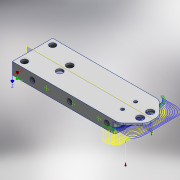
# Autodesk Inventor part: c-head-flange
Saved by Autodesk Inventor 2016 (Build 200138000, 138)
## iProperties
Created: 2015-05-12
Part Number: c-head-flange
Material: Aluminum 6061
Document SubType Name: Modeling
Designer: as
Mass: 10.115 g
Surface Area: 39.4991 cm^2
Volume: 3.74628 cm^3
Density: 2.7 g/cm^3
Appearance: Aluminum - Flat
Author: as
Autodesk Inventor part; units mm, degrees
ref_plane "YZ Plane" through (0, 0, 0) normal (1, 0, 0) x (0, 1, 0)
ref_plane "XZ Plane" through (0, 0, 0) normal (0, 1, 0) x (-1, 0, 0)
ref_plane "XY Plane" through (0, 0, 0) normal (0, 0, 1) x (1, 0, 0)
sketch "Sketch1" plane through (0, 0, 0) normal (0, 0, 1) x (1, 0, 0)
  line L0 (-6, -20) -> (60, -20)
  line L1 (60, -20) -> (60, 0)
  line L2 (60, 0) -> (-6, 0)
  line L3 (-6, 0) -> (-6, -20)
  point P0 (0, 0)
  dimension "d2" = 20
  dimension "d3" = 66
  dimension "d8" = 60
  dimension "d9" = 0
  constraints: 8 end point, 2 parallel, 1 horizontal, 1 perpendicular
  measures "d2" distance of L0.end L1.end
  measures "d3" distance of L1.end L2.end
  measures "d8" distance from line of point (0, 0) L1
  measures "d9" distance from line of point (0, 0) L2
extrude "Extrusion1" add sketch "Sketch1" along normal blind 6
sketch "Sketch5" plane through (0, 0, 6) normal (0, 0, 1) x (1, 0, 0)
  line L0 (-6, 0) -> (-6, -20) projected
  point P0 (0, 0)
  point P1 (-3, -3)
  point P2 (-3, -17)
  dimension "d48" = 3
  dimension "d50" = 17
  dimension "d51" = 3
  dimension "d53" = 3
  measures "d48" horizontal distance of L0.start point (-3, -3)
  measures "d50" vertical distance of L0.start point (-3, -17)
  measures "d51" distance from line of L0 point (-3, -3)
  measures "d53" distance from line of L0 point (-3, -17)
hole "Hole6" at (-3, -3, 6) at (-3, -17, 6) direction (0, 0, -1) diameter 3 end through all
sketch "Sketch7" plane through (0, 0, 0) normal (0, 0, -1) x (-1, 0, 0)
  line L0 (-60, 0) -> (0, 0) projected
  line L1 (6, 0) -> (6, -20) projected
  line L2 (-60, -20) -> (-60, 0) projected
  point P0 (-42, -6.75)
  point P1 (-42, -13.25)
  dimension "d68" = 6.75
  dimension "d70" = 6.5
  dimension "d207" = 18
  constraints: 1 vertical alignment
  measures "d68" distance from line of L0 point (-42, -6.75)
  measures "d70" distance of point (-42, -13.25) point (-42, -6.75)
  measures "d207" distance from line of L2 point (-42, -13.25)
hole "Hole9" at (42, -13.25, 0) at (42, -6.75, 0) direction (0, 0, 1) diameter 1.567 end through all thread size "M2x0.4" class "6H" standard "ISO Metric profile"
sketch "Sketch8" plane through (0, 0, 0) normal (0, 0, -1) x (-1, 0, 0)
  line L0 (-35.9, -15.5) -> (-1, -15.5)
  line L1 (-1, -4.5) -> (-35.9, -4.5)
  line L2 (1, -6.5) -> (1, -13.5)
  arc A0 (-1, -15.5) -> (1, -13.5) centre (-1, -13.5) ccw
  arc A1 (1, -6.5) -> (-1, -4.5) centre (-1, -6.5) ccw
  line L3 (-60, 0) -> (6, 0) projected
  line L4 (6, -20) -> (-60, -20) projected
  line L5 (6, -20) -> (-60, -20) projected
  line L6 (-39, -12.4) -> (-39, -7.6)
  arc A2 (-39, -12.4) -> (-35.9, -15.5) centre (-35.9, -12.4) ccw
  arc A3 (-35.9, -4.5) -> (-39, -7.6) centre (-35.9, -7.6) ccw
  line L7 (6, 0) -> (6, -20) projected
  line L8 (-60, -20) -> (-60, 0)
  line L9 (-60, 0) -> (-45, 0)
  line L10 (-45, 0) -> (-45, -20)
  line L11 (-45, -20) -> (-60, -20)
  point P0 (-39, -15.5)
  point P1 (-39, -4.5)
  dimension "d149" = 2
  dimension "d166" = 4.5
  dimension "d167" = 4.5
  dimension "d168" = 66
  dimension "d203" = 3.1
  dimension "d204" = 5
  dimension "d205" = 45
  dimension "d214" = 15
  constraints: 16 end point, 8 point on circle, 8 tangent, 4 centre point, 4 point on line, 3 parallel, 2 equal radius, 2 perpendicular, 2 vertical
  measures "d149" radius of A0
  measures "d166" distance between parallel lines of L3 L1
  measures "d167" distance between parallel lines of L4 L0
  measures "d168" distance of L3.start L3.end
  measures "d203" radius of A2
  measures "d204" distance between parallel lines of L7 L2
  measures "d205" distance between parallel lines of L7 L6
  measures "d214" distance of L3.start L9.end
extrude "Extrusion2" cut sketch "Sketch8" against normal blind 5 contours A2 L6 A3 L1 A1 L2 A0 L0 | L3 L10 L4 L8
ref_plane "Work Plane1" through (-6, -10, 0) normal (0, 1, 0) x (1, 0, 0)
sketch "Sketch6" plane through (-6, -20, 0) normal (0, -1, 0) x (1, 0, 0)
  point P0 (43, 3)
  point P1 (30, 3)
  point P2 (17, 3)
sketch "Sketch11" plane through (0, 0, 5) normal (0, 0, -1) x (-1, 0, 0)
  point P0 (-10, -12.5)
hole "Hole12" at (10, -12.5, 5) direction (0, 0, 1) diameter 3.2 depth 1
sketch "Sketch13" plane through (-5.75, -20, 0) normal (0, -1, 0) x (1, 0, 0)
  point P0 (46.75, 3)
  point P1 (28.25, 3)
  point P2 (9.75, 3)
sketch "Sketch14" plane through (0, 0, 5) normal (0, 0, -1) x (-1, 0, 0)
  point P0 (-50, -12.5)
hole "Hole18" at (50, -12.5, 5) direction (0, 0, 1) diameter 3.4 depth 1
sketch "Sketch4" plane through (-6, -20, 0) normal (0, -1, 0) x (1, 0, 0)
  line L0 (6, 0) -> (66, 0) projected
  line L1 (0, 0) -> (0, 6) projected
  point P0 (10, 3)
  point P1 (28.5, 3)
  point P2 (47, 3)
  dimension "d42" = 4
  dimension "d43" = 22.5
  dimension "d44" = 41
  dimension "d45" = 3
  dimension "d46" = 3
  dimension "d47" = 3
  dimension "d146" = 6
  measures "d42" horizontal distance of L0.start point (10, 3)
  measures "d43" horizontal distance of point (28.5, 3) L0.start
  measures "d44" horizontal distance of L0.start point (47, 3)
  measures "d45" vertical distance of point (10, 3) L0.start
  measures "d46" distance from line of L0 point (28.5, 3)
  measures "d47" distance from line of L0 point (47, 3)
  measures "d146" distance from line of L1 L0.start
hole "Hole5" at (41, -20, 3) at (22.5, -20, 3) at (4, -20, 3) direction (0, 1, 0) diameter 2.459 end through all thread size "M3x0.5" class "6H" standard "ISO Metric profile"
mirror "Mirror3" about plane through (-6, -10, 0) normal (0, 1, 0) of "Hole12", "Hole18"
move faces "Move1" translate (-6, 0, 0) faces at (60, -13.3333, 5.3333)
chamfer "Chamfer1" distance 7 angle 45 2 edges at (54, 0, 5.5) (54, -20, 5.5)
fillet "Fillet4" radius 4 4 edges at (54, -13, 5.5) (47, -20, 5.5) (54, -7, 5.5) (47, 0, 5.5)
fillet "Fillet5" radius 1 2 edges at (45, 0, 2.5) (45, -20, 2.5)
chamfer "Chamfer2" distance 0.5 angle 45 8 edges at (18.45, -15.5, 0) (38.092, -14.592, 0) (39, -10, 0) (38.092, -5.408, 0) (18.45, -4.5, 0) (-0.4142, -5.0858, 0) (-1, -10, 0) (-0.4142, -14.9142, 0)
equation "\"d3\" = d0"
equation "\"d53\" = d51"
equation "\"d167\" = d166"
equation "\"d43\" = 0.5 * d44 + 0.5 * d42"
equation "\"d46\" = d45"
equation "\"d47\" = d45"
equation "\"d36\" = d2"
equation "\"d0\" = 66"
body "Solid1"
